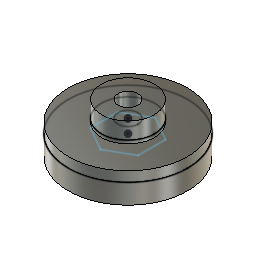
design (Autodesk Fusion 360 design; units mm, degrees)
Autodesk Fusion 360 part; units mm, degrees
sketch "Sketch1" plane through (0, 0, 0) normal (0, 0, 1) x (1, 0, 0) in component "Component'"
  line L0 (3.6, 2.0785) -> (0, 4.1569)
  line L1 (0, 4.1569) -> (-3.6, 2.0785)
  line L2 (-3.6, 2.0785) -> (-3.6, -2.0785)
  line L3 (-3.6, -2.0785) -> (0, -4.1569)
  line L4 (0, -4.1569) -> (3.6, -2.0785)
  line L5 (3.6, -2.0785) -> (3.6, 2.0785)
  circle A0 centre (0, 0) radius 9
  dimension "d1" = 3.6
  dimension "d2" = 18
  constraint coincident A0.centre origin
  measures "d1" distance of A0.centre L5
  measures "d2" diameter of A0
extrude "Extrude3" add sketch "Sketch1" along normal blind 1.5 contours L0 L1 L2 L3 L4 L5 | A0 makes body 1 in component "Component'"
extrude "Extrude1" add sketch "Sketch1" against normal blind 3 separate body makes body 2 in component "Component'"
ref_plane "WorkPlane1" through (0, 0, 2) normal (0, 0, 1) x (1, 0, 0) in component "Component'"
sketch "Sketch2" plane through (0, 0, 2) normal (0, 0, 1) x (1, 0, 0) in component "Component'"
  circle A0 centre (0, 0) radius 1.5
  circle A1 centre (0, 0) radius 4
  dimension "d6" = 3
  dimension "d7" = 8
  constraint coincident A0.centre A1.centre
  measures "d6" diameter of A0
  measures "d7" diameter of A1
extrude "Extrude2" add sketch "Sketch2" along normal blind 2.5 and the other way blind 0.5 separate body makes body 3 in component "Component'"
loft "Loft3" cut profiles "Sketch1", "Sketch2" section 1 contours L0 L1 L2 L3 L4 L5 section 2 contours A0 bodies 1 3 in component "Component'"
sketch "Sketch3" plane through (0, 0, 0) normal (0, 1, 0) x (1, 0, 0) in component "Component'"
  line L0 (0, -6) -> (0, 0) construction
  constraint coincident L0.end origin
  constraint vertical L0
component "Component'" placed x (1, 0, 0) y (0, 1, 0) z (0, 0, 1) at (0, 0, 0)
